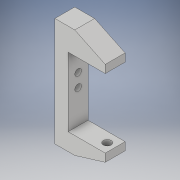
# Autodesk Inventor part: clamp
Saved by Autodesk Inventor 2019.3 (Build 233278000, 278)
## iProperties
Created: 2019-04-14
Part Number: clamp
Material: Generic
Document SubType Name: Modeling
Designer: peter
Density: 1 g/cm^3
Appearance: Default
Author: peter
Autodesk Inventor part; units mm, degrees
ref_plane "YZ Plane" through (0, 0, 0) normal (1, 0, 0) x (0, 1, 0)
ref_plane "XZ Plane" through (0, 0, 0) normal (0, 1, 0) x (-1, 0, 0)
ref_plane "XY Plane" through (0, 0, 0) normal (0, 0, 1) x (1, 0, 0)
sketch "Sketch1" plane through (0, 0, 0) normal (0, 0, 1) x (1, 0, 0)
  line L0 (0, 0) -> (0, -82)
  line L1 (0, -82) -> (15, -82)
  line L2 (15, -82) -> (15, -75) construction
  line L3 (15, -75) -> (38, -75) construction
  line L4 (15, -82) -> (38, -75)
  line L5 (38, -75) -> (38, -69)
  line L6 (38, -69) -> (10, -69)
  line L7 (10, -69) -> (10, -17)
  line L8 (10, -17) -> (38, -17)
  line L9 (38, -17) -> (38, -11)
  line L10 (0, 0) -> (15, 0)
  line L11 (15, 0) -> (38, -11)
  dimension "d0" = 82
  dimension "d1" = 15
  dimension "d2" = 90
  dimension "d3" = 7
  dimension "d4" = 23
  dimension "d5" = 6
  dimension "d6" = 28
  dimension "d7" = 90
  dimension "d8" = 52
  dimension "d9" = 90
  dimension "d10" = 28
  dimension "d11" = 6
  dimension "d12" = 15
  constraints: 24 end point, 4 perpendicular, 3 vertical, 2 point on line, 1 horizontal
  measures "d0" distance of L0.start L0.end
  measures "d1" distance of L0.end L1.end
  measures "d2" angle of L1 L0
  measures "d3" distance of L1.end L2.end
  measures "d4" distance of L2.end L3.end
  measures "d5" distance of L3.end L5.end
  measures "d6" distance of L5.end L6.end
  measures "d7" angle of L6 L5
  measures "d8" distance of L6.end L7.end
  measures "d9" angle of L6 L7
  measures "d10" distance of L7.end L8.end
  measures "d11" distance of L8.end L9.end
  measures "d12" distance of L0.start L10.end
extrude "Extrusion1" add sketch "Sketch1" along normal blind 15
sketch "Sketch2" plane through (10, -69, 0) normal (0, 1, 0) x (1, 0, 0)
  line L0 (5, 0) -> (28, 0) projected
  line L1 (28, 0) -> (28, -15) projected
  line L2 (5, -15) -> (28, -15) projected
  line L3 (5, 0) -> (5, -15) projected
  line L4 (28, 0) -> (28, -15) construction
  line L5 (28, -7.5) -> (22, -7.5) construction
  circle A0 centre (22, -7.5) radius 3
  point P0 (-10, 0)
  dimension "d15" = 6
  dimension "d16" = 6
  constraints: 2 end point, 1 centre point, 1 coincident, 1 horizontal, 1 midpoint
  measures "d15" distance of L5.start L5.end
  measures "d16" diameter of A0
extrude "Extrusion2" cut sketch "Sketch2" against normal blind 15 contours A0
sketch "Sketch3" plane through (10, -69, 0) normal (1, 0, 0) x (0, 0, -1)
  line L0 (0, 52) -> (-15, 52) construction
  line L1 (-7.5, 52) -> (-7.5, 35) construction
  line L2 (-7.5, 52) -> (9.5, 52) construction
  line L3 (-7.5, 35) -> (-7.5, 25) construction
  circle A0 centre (-7.5, 35) radius 2.5
  circle A1 centre (-7.5, 25) radius 2.5
  point P0 (0, 69)
  dimension "d19" = 17
  dimension "d20" = 90
  dimension "d21" = 10
  dimension "d22" = 5
  dimension "d23" = 5
  constraints: 6 end point, 2 centre point, 2 coincident, 2 vertical, 1 horizontal, 1 midpoint, 1 perpendicular
  measures "d19" distance of L1.start L1.end
  measures "d20" angle of L1 L2
  measures "d21" distance of L1.end L3.end
  measures "d22" diameter of A0
  measures "d23" diameter of A1
extrude "Extrusion3" cut sketch "Sketch3" against normal blind 15
body "Solid1"
